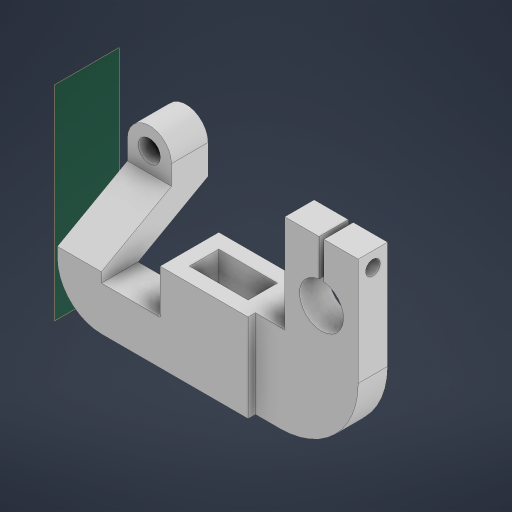
# Autodesk Inventor part: Część17
Saved by Autodesk Inventor 2023 (Build 270158000, 158)
## iProperties
Created: 2023-05-08
Part Number: Część17
Material: Ogólny
Document SubType Name: Modeling
Designer: Adam
Density: 1 g/cm^3
Appearance: Domyślna
Author: Adam
Autodesk Inventor part; units mm, degrees
ref_plane "YZ Plane" through (0, 0, 0) normal (1, 0, 0) x (0, 1, 0)
ref_plane "XZ Plane" through (0, 0, 0) normal (0, 1, 0) x (-1, 0, 0)
ref_plane "XY Plane" through (0, 0, 0) normal (0, 0, 1) x (1, 0, 0)
sketch "Szkic1" plane through (0, 0, 0) normal (0, 0, 1) x (1, 0, 0)
  line L0 (0, 0) -> (36, 0)
  line L1 (36, 0) -> (36, 36)
  line L2 (36, 36) -> (0, 36)
  line L3 (0, 36) -> (0, 0)
  line L4 (0, 0) -> (-24, 0)
  line L5 (-42, 18) -> (-42, 18)
  line L6 (-42, 18) -> (0, 18)
  line L7 (0, 18) -> (0, 0)
  line L8 (36, 36) -> (78, 36)
  line L9 (78, 36) -> (78, 32)
  line L10 (46, 0) -> (36, 0)
  line L11 (36, 0) -> (36, 36)
  line L12 (78, 36) -> (48, 36)
  line L13 (48, 36) -> (48, 76)
  line L14 (48, 76) -> (78, 76)
  line L15 (78, 76) -> (78, 36)
  arc A0 (46, 0) -> (78, 32) centre (46, 32) ccw
  arc A1 (-42, 18) -> (-24, 0) centre (-24, 18) ccw
  point P0 (-42, 0)
  point P1 (78, 0)
  dimension "d0" = 36
  dimension "d1" = 36
  dimension "d2" = 42
  dimension "d3" = 18
  dimension "d4" = 42
  dimension "d5" = 30
  dimension "d6" = 40
  dimension "d7" = 32
  dimension "d8" = 18
  constraints: 32 end point, 8 parallel, 4 horizontal, 4 perpendicular, 4 point on circle, 4 point on line, 4 tangent, 2 centre point
  measures "d0" distance of L2.end L1.end
  measures "d1" distance of L1.end L0.end
  measures "d2" distance of L5.end L6.end
  measures "d3" distance of point (-42, 0) L5.end
  measures "d4" distance of point (78, 0) L10.end
  measures "d5" distance of L13.end L14.end
  measures "d6" distance of L12.end L13.end
  measures "d7" radius of A0
  measures "d8" radius of A1
extrude "Wyciągnięcie proste1" add sketch "Szkic1" against normal blind 24
sketch "Szkic2" plane through (0, 0, 0) normal (0, 0, 1) x (1, 0, 0)
  line L0 (78, 76) -> (78, 32) projected
  line L1 (46, 0) -> (-24, 0) projected
  line L2 (78, 76) -> (36, 76)
  line L3 (36, 76) -> (36, 0)
  line L4 (36, 0) -> (78, 0)
  line L5 (78, 0) -> (78, 76)
  point P0 (0, 0)
  constraints: 8 end point, 2 parallel, 1 horizontal, 1 perpendicular, 1 point on line
extrude "Wyciągnięcie proste2" cut sketch "Szkic2" against normal blind 3
sketch "Szkic3" plane through (0, 0, -24) normal (0, 0, -1) x (-1, 0, 0)
  line L0 (-48, 76) -> (-78, 76) projected
  line L1 (-46, 0) -> (-36, 0) projected
  line L2 (-78, 76) -> (-36, 76)
  line L3 (-36, 76) -> (-36, 0)
  line L4 (-36, 0) -> (-78, 0)
  line L5 (-78, 0) -> (-78, 76)
  line L6 (0, 36) -> (0, 18) projected
  line L7 (0, 36) -> (42, 36)
  line L8 (42, 36) -> (42, 0)
  line L9 (42, 0) -> (0, 0)
  line L10 (0, 0) -> (0, 36)
  point P0 (0, 0)
  constraints: 16 end point, 4 parallel, 2 horizontal, 2 perpendicular, 1 point on line
extrude "Wyciągnięcie proste3" cut sketch "Szkic3" against normal blind 9 contours L2 L3 L1 L4 L5 L0
sketch "Szkic4" plane through (0, 0, -24) normal (0, 0, -1) x (-1, 0, 0)
  line L0 (42, 18) -> (0, 18) projected
  line L1 (0, 0) -> (42, 0)
  line L2 (42, 0) -> (42, 18)
  line L3 (42, 18) -> (0, 18)
  line L4 (0, 18) -> (0, 0)
  constraints: 8 end point, 2 parallel, 1 horizontal, 1 perpendicular
extrude "Wyciągnięcie proste4" cut sketch "Szkic4" against normal blind 9
ref_plane "Płaszczyzna konstrukcyjna1" through (-42, 18, 0) normal (-1, 0, 0) x (0, -1, 0)
sketch "Szkic5" plane through (-42, 18, 0) normal (-1, 0, 0) x (0, -1, 0)
  line L0 (0, 0) -> (0, -15) projected
  line L1 (-18, -15) -> (18, -15) projected
  line L2 (0, -15) -> (-16, -43.6236)
  line L3 (-16, -43.6236) -> (-37, -43.6236)
  line L4 (-37, -43.6236) -> (-37, -28.6236)
  line L5 (-37, -28.6236) -> (-20, -28.6236)
  line L6 (-20, -28.6236) -> (-4, 0)
  line L7 (-18, 0) -> (0, 0) projected
  line L8 (0, 0) -> (0, -15)
  point P0 (18, 0)
  point P1 (-28.5, -28.6236)
  dimension "d17" = 16
  dimension "d18" = 15
  dimension "d19" = 4
  dimension "d20" = 16
  dimension "d21" = 21
  constraints: 12 end point, 2 midpoint, 2 perpendicular, 1 collinear, 1 horizontal, 1 point on line
  measures "d17" horizontal distance of L2.start L2.end
  measures "d18" distance from line of point (-28.5, -28.624) L3
  measures "d19" distance of L0.start L6.end
  measures "d20" horizontal distance of L6.end L5.end
  measures "d21" distance from line of L4 L2.end
extrude "Wyciągnięcie proste5" add sketch "Szkic5" against normal blind 18
full round fillet "Zaokrąglenie pełne1" first side at (-24, 26, -14.5412) centre faces at (-36, 55, -33.6236) second side at (-42, 26, -14.5412)
sketch "Szkic6" plane through (-42, 38, -28.6236) normal (0, 0, 1) x (1, 0, 0)
  arc A0 (18, 8) -> (0, 8) centre (9, 8) ccw projected
  point P0 (42, -38)
  constraints: 1 coincident
hole "Otwór1" at (-33, 46, -28.6236) direction (0, 0, -1) diameter 9 end through all
sketch "Szkic7" plane through (48, 36, -3) normal (-1, 0, 0) x (0, 0, 1)
  point P0 (3, -36)
  point P1 (-6, 34)
hole "Otwór2" at (48, 70, -9) direction (1, 0, 0) diameter 6 end through all
sketch "Szkic8" plane through (0, 0, -3) normal (0, 0, 1) x (1, 0, 0)
  point P0 (0, 0)
  point P1 (63, 52)
hole "Otwór3" at (63, 52, -3) direction (0, 0, -1) diameter 18 end through all
sketch "Szkic9" plane through (48, 76, -3) normal (0, 1, 0) x (1, 0, 0)
  line L0 (0, 0) -> (30, 0) projected
  line L1 (14, 12) -> (16, 12)
  line L2 (16, 12) -> (16, 0)
  line L3 (16, 0) -> (14, 0)
  line L4 (14, 0) -> (14, 12)
  line L5 (30, 0) -> (30, 12) projected
  point P0 (-48, -3)
  point P1 (14, 0)
  dimension "d45" = 2
  dimension "d46" = 14
  constraints: 8 end point, 2 parallel, 1 horizontal, 1 perpendicular, 1 point on line
  measures "d45" distance of L2.end L3.end
  measures "d46" distance between parallel lines of L5 L2
extrude "Wyciągnięcie proste6" cut sketch "Szkic9" against normal up to surface
sketch "Szkic10" plane through (0, 36, 0) normal (0, 1, 0) x (1, 0, 0)
  line L0 (6, 18) -> (30, 18)
  line L1 (30, 18) -> (30, 6)
  line L2 (30, 6) -> (6, 6)
  line L3 (6, 6) -> (6, 18)
  line L4 (0, 24) -> (36, 24) projected
  line L5 (0, 0) -> (0, 24) projected
  point P0 (6, 12)
  dimension "d49" = 24
  dimension "d50" = 12
  dimension "d51" = 6
  dimension "d52" = 6
  constraints: 8 end point, 2 parallel, 1 horizontal, 1 midpoint, 1 perpendicular
  measures "d49" distance from line of L1 point (6, 12)
  measures "d50" distance between parallel lines of L2 L0
  measures "d51" distance between parallel lines of L4 L0
  measures "d52" distance between parallel lines of L5 L3
extrude "Wyciągnięcie proste7" cut sketch "Szkic10" against normal through all
